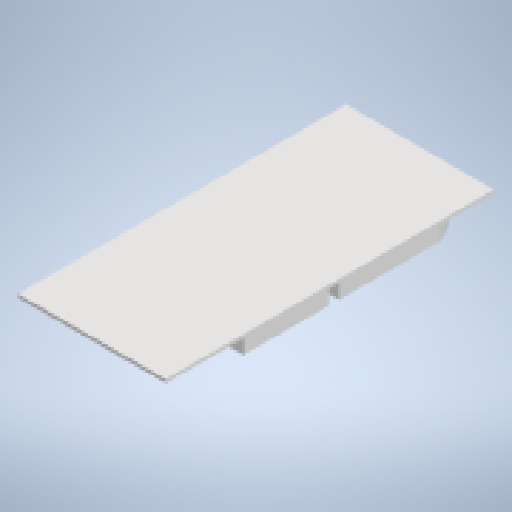
# Autodesk Inventor part: sole_paint_support_base
Saved by Autodesk Inventor 2026.1 (Build 301233020, 233B)
## iProperties
Created: 2026-02-24
Part Number: sole_paint_support_base
Material: 一般
Document SubType Name: Modeling
Designer: hibik
Density: 1 g/cm^3
Appearance: 既定
Author: hibik
Autodesk Inventor part; units mm, degrees
ref_plane "YZ Plane" through (0, 0, 0) normal (1, 0, 0) x (0, 1, 0)
ref_plane "XZ Plane" through (0, 0, 0) normal (0, 1, 0) x (-1, 0, 0)
ref_plane "XY Plane" through (0, 0, 0) normal (0, 0, 1) x (1, 0, 0)
sketch "スケッチ1" plane through (0, 0, 0) normal (0, 1, 0) x (-1, 0, 0)
  line L0 (-21, 51.2893) -> (-21, -42) projected
  line L1 (-21, -42) -> (21, -42) projected
  line L2 (21, -42) -> (21, 51.2893) projected
  line L3 (-21, 51.2893) -> (21, 51.2893) projected
  line L4 (-19.7, 0.7) -> (19.7, 0.7) projected
  line L5 (19.7, 0.7) -> (19.7, -28.3561) projected
  arc A0 (8.8769, -40.7) -> (19.7, -28.3561) centre (0, -22) ccw projected
  line L6 (8.8769, -40.7) -> (-8.8769, -40.7) projected
  arc A1 (-19.7, -28.3561) -> (-8.8769, -40.7) centre (0, -22) ccw projected
  line L7 (-19.7, -28.3561) -> (-19.7, 0.7) projected
  line L8 (-19.7, 2.3) -> (-19.7, 33.1604) projected
  ellipse E0 centre (-12, 33.1604) end of major axis (-12, 25.3416) minor radius 7.7 (-19.3049, 35.6329) -> (-19.7, 33.1604) ccw projected
  line L9 (-16.2595, 44.9098) -> (-19.3049, 35.6329) projected
  ellipse E1 centre (-8.9547, 42.4373) end of major axis (-8.9547, 34.6185) minor radius 7.7 (-8.9547, 50.2561) -> (-16.2595, 44.9098) ccw projected
  line L10 (8.9547, 50.2561) -> (-8.9547, 50.2561) projected
  ellipse E2 centre (8.9547, 42.4373) end of major axis (8.9547, 34.6185) minor radius 7.7 (16.2595, 44.9098) -> (8.9547, 50.2561) ccw projected
  line L11 (19.3049, 35.6329) -> (16.2595, 44.9098) projected
  ellipse E3 centre (12, 33.1604) end of major axis (12, 25.3416) minor radius 7.7 (19.7, 33.1604) -> (19.3049, 35.6329) ccw projected
  line L12 (19.7, 33.1604) -> (19.7, 2.3) projected
  line L13 (19.7, 2.3) -> (-19.7, 2.3) projected
  line L14 (8.9547, 49.6561) -> (-8.9547, 49.6561)
  line L15 (-15.6895, 44.7227) -> (-18.7348, 35.4458)
  line L16 (-19.1, 33.1604) -> (-19.1, 2.9)
  line L17 (-19.1, 2.9) -> (19.1, 2.9)
  line L18 (19.1, 2.9) -> (19.1, 33.1604)
  line L19 (18.7348, 35.4458) -> (15.6895, 44.7227)
  line L20 (19.1, -28.261) -> (19.1, 0.1)
  line L21 (19.1, 0.1) -> (-19.1, 0.1)
  line L22 (-19.1, 0.1) -> (-19.1, -28.261)
  arc A2 (-19.1, -28.261) -> (-8.7407, -40.1) centre (0, -22) ccw
  line L23 (-8.7407, -40.1) -> (8.7407, -40.1)
  arc A3 (8.7407, -40.1) -> (19.1, -28.261) centre (0, -22) ccw
  line L24 (19.1, 27.3) -> (-19.1, 27.3)
  point P0 (0, 0)
  dimension "d0" = 0.6
  dimension "d1" = 0.6
  dimension "d2" = 25
  constraints: 22 end point, 7 parallel, 4 point on circle, 2 centre point, 2 point on line, 1 perpendicular, 23 other
  measures "d0" distance between parallel lines of L11 L19
  measures "d1" distance between parallel lines of L5 L20
  measures "d2" distance between parallel lines of L13 L24
extrude "押し出し1" add sketch "スケッチ1" against normal blind 6 contours L24 L18 L17 L16 | A3 L23 A2 L22 L21 L20
sketch "スケッチ2" plane through (0, 0, 0) normal (0, 1, 0) x (1, 0, 0)
  line L0 (21, -51.2893) -> (21, 42) projected
  line L1 (21, 42) -> (-21, 42) projected
  line L2 (-21, 42) -> (-21, -51.2893) projected
  line L3 (21, -51.2893) -> (-21, -51.2893) projected
  line L4 (19.7, -0.7) -> (-19.7, -0.7) projected
  line L5 (-19.7, -0.7) -> (-19.7, 28.3561) projected
  arc A0 (-8.8769, 40.7) -> (-19.7, 28.3561) centre (0, 22) ccw projected
  line L6 (-8.8769, 40.7) -> (8.8769, 40.7) projected
  arc A1 (19.7, 28.3561) -> (8.8769, 40.7) centre (0, 22) ccw projected
  line L7 (19.7, 28.3561) -> (19.7, -0.7) projected
  line L8 (19.7, -2.3) -> (19.7, -33.1604) projected
  ellipse E0 centre (12, -33.1604) end of major axis (12, -25.3416) minor radius 7.7 (19.3049, -35.6329) -> (19.7, -33.1604) ccw projected
  line L9 (16.2595, -44.9098) -> (19.3049, -35.6329) projected
  ellipse E1 centre (8.9547, -42.4373) end of major axis (8.9547, -34.6185) minor radius 7.7 (8.9547, -50.2561) -> (16.2595, -44.9098) ccw projected
  line L10 (-8.9547, -50.2561) -> (8.9547, -50.2561) projected
  ellipse E2 centre (-8.9547, -42.4373) end of major axis (-8.9547, -34.6185) minor radius 7.7 (-16.2595, -44.9098) -> (-8.9547, -50.2561) ccw projected
  line L11 (-19.3049, -35.6329) -> (-16.2595, -44.9098) projected
  ellipse E3 centre (-12, -33.1604) end of major axis (-12, -25.3416) minor radius 7.7 (-19.7, -33.1604) -> (-19.3049, -35.6329) ccw projected
  line L12 (-19.7, -33.1604) -> (-19.7, -2.3) projected
  line L13 (-19.7, -2.3) -> (19.7, -2.3) projected
  point P0 (0, 0)
  constraints: 4 other
extrude "押し出し2" add sketch "スケッチ2" along normal blind 1 contours L3 L2 L1 L0 | L4 L5 A0 L6 A1 L7 | L8 E0 L9 E1 L10 E2 L11 E3 L12 L13
